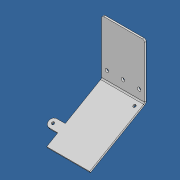
# Autodesk Inventor part: Fan_Holder
Saved by Autodesk Inventor 2020 (Build 240168000, 168)
## iProperties
Created: 2021-06-06
Part Number: Fan_Holder
Material: 一般
Document SubType Name: Sheet Metal
Designer: ken113
Density: 1 g/cm^3
Sheet Metal Rule: Default_mm
Appearance: 既定
Author: ken113
Autodesk Inventor part; units mm, degrees
ref_plane "YZ Plane" through (0, 0, 0) normal (1, 0, 0) x (0, 1, 0)
ref_plane "XZ Plane" through (0, 0, 0) normal (0, 1, 0) x (-1, 0, 0)
ref_plane "XY Plane" through (0, 0, 0) normal (0, 0, 1) x (1, 0, 0)
sketch "スケッチ1" plane through (0, 0, 0) normal (0, 0, 1) x (1, 0, 0)
  line L0 (20, 0) -> (-20, 0)
  line L1 (-20, 0) -> (-20, 50)
  line L2 (-20, 50) -> (20, 50)
  line L3 (20, 50) -> (20, 0)
  line L4 (20, 0) -> (-20, 50) construction
  line L5 (-20, 0) -> (20, 50) construction
  point P0 (0, 0)
  point P1 (0, 25)
  point P2 (0, 0)
  point P3 (0, 25)
  dimension "d0" = 40
  dimension "d1" = 50
  measures "d0" distance of L1.end L2.end
  measures "d1" distance of L0.end L1.end
extrude "プレート1" add sketch "スケッチ1" along normal blind 1.6
sketch "スケッチ2" plane through (20, -1.3856, 2.4) normal (0, -0.8660254, -0.5) x (1, 0, 0)
  line L0 (-40, 0) -> (0, 0)
  line L1 (0, 0) -> (0, 57.9525)
  line L2 (0, 57.9525) -> (-40, 57.9525)
  line L3 (-40, 57.9525) -> (-40, 0)
  constraints: 6 end point, 1 horizontal, 1 perpendicular, 1 vertical
edge flange "フランジ1" height 59.8 angle 60 thickness 1.6 bend radius 1.6 thickness toward (0, -0.8660254, -0.5) relief straight relief width 1.6 relief depth 0.8 edges at (0, 0, 1.6) wall of the first edge with corners at (-20, -1.3856, 2.4) (20, -1.3856, 2.4) (20, -30.3619, 52.5883) (-20, -30.3619, 52.5883)
bend "曲げ1"
corner "コーナー1"
sketch "スケッチ3" plane through (0, 0, 0) normal (0, 0, -1) x (-1, 0, 0)
  line L0 (-20, 0) -> (20, 0) projected
  line L1 (20, 0) -> (20, 50) projected
  line L2 (20, 50) -> (-20, 50) projected
  line L3 (-20, 50) -> (-20, 0) projected
  point P0 (0, 0)
  point P1 (-15, 8)
  point P2 (15, 8)
  point P3 (0, 8)
  point P4 (0, 0)
  dimension "d14" = 5
  dimension "d15" = 5
  dimension "d62" = 8
  constraints: 2 horizontal alignment, 1 midpoint, 1 vertical alignment
  measures "d14" distance from line of point (-15, 8) L3
  measures "d15" distance from line of L1 point (15, 8)
  measures "d62" distance from line of point (-15, 8) L0
hole "穴1" at (15, 8, 0) at (-15, 8, 0) at (0, 8, 0) direction (0, 0, 1) diameter 3.2 depth 1.6 tip angle 118
sketch "スケッチ4" plane through (-20, -31.7475, 51.7883) normal (0, -0.8660254, -0.5) x (1, 0, 0)
  line L0 (0, -57.9525) -> (40, -57.9525) projected
  line L1 (40, 0) -> (40, -57.9525) projected
  line L2 (0, 0) -> (40, 0) projected
  line L3 (0, -57.9525) -> (0, 0) projected
  point P0 (20, -60.7238)
  point P1 (35, -53.9525)
  dimension "d23" = 5
  dimension "d24" = 4
  measures "d23" distance from line of point (35, -53.952) L1
  measures "d24" distance from line of L0 point (35, -53.952)
hole "穴2" at (15, -4.7713, 5.0641) direction (0, 0.8660254, 0.5) diameter 2.459 end through all thread size "M3x0.5" class "6H" standard "ISO Metric profile"
sketch "スケッチ5" plane through (-20, -31.7475, 51.7883) normal (0, -0.8660254, -0.5) x (1, 0, 0)
  circle A0 centre (35, -53.9525) radius 1.2295 projected
  line L0 (0, 0) -> (0, -57.9525) projected
  line L1 (0, -11.9525) -> (-12, -11.9525)
  line L2 (-12, -11.9525) -> (-12, -19.9525)
  line L3 (-12, -19.9525) -> (0, -19.9525)
  line L4 (0, -19.9525) -> (0, -11.9525)
  point P0 (20, -60.7238)
  point P1 (-8, -15.9525)
  point P2 (0, -19.9525)
  dimension "d32" = 43
  dimension "d33" = 38
  dimension "d34" = 4
  dimension "d35" = 8
  dimension "d36" = 4
  constraints: 8 end point, 2 parallel, 1 horizontal, 1 perpendicular, 1 point on line
  measures "d32" horizontal distance of point (-8, -15.952) A0.centre
  measures "d33" vertical distance of point (-8, -15.952) A0.centre
  measures "d34" distance from line of point (-8, -15.952) L1
  measures "d35" distance of L1.end L2.end
  measures "d36" distance from line of point (-8, -15.952) L2
extrude "押し出し1" add sketch "スケッチ5" against normal up to surface (1.6 mm away) contours L0 L3 L2 L1
sketch "スケッチ6" plane through (-20, -31.7475, 51.7883) normal (0, -0.8660254, -0.5) x (1, 0, 0)
  circle A0 centre (35, -53.9525) radius 1.2295 projected
  point P0 (20, -60.7238)
  point P1 (-8, -15.9525)
  dimension "d39" = 43
  dimension "d40" = 38
  measures "d39" horizontal distance of point (-8, -15.952) A0.centre
  measures "d40" vertical distance of point (-8, -15.952) A0.centre
hole "穴3" at (-28, -23.7713, 37.9731) direction (0, 0.8660254, 0.5) diameter 2.459 depth 8.8 tip angle 118 thread size "M3x0.5" class "6H" standard "ISO Metric profile"
fillet "フィレット1" radius 4 2 edges at (-32, -21.0785, 34.909) (-32, -25.0785, 41.8372)
fillet "フィレット2" radius 2 2 edges at (20, 50, 0.8) (-20, 50, 0.8)
equation "\"d21\" = Thickness"
equation "\"d30\" = Thickness"
equation "\"d2\" = Thickness"
equation "\"d3\" = BendReliefWidth"
equation "\"d4\" = BendReliefDepth"
equation "\"d5\" = MinimumRemnant"
equation "\"d6\" = TransitionRadius"
equation "\"d9\" = BendRadius"
equation "\"d10\" = CornerReliefSize"
equation "\"d11\" = GapSize"
equation "\"d12\" = JacobiRadiusSize"
equation "\"BendRadius\" = Thickness"
equation "\"BendReliefWidth\" = Thickness"
equation "\"BendReliefDepth\" = 0.5 * Thickness"
equation "\"CornerReliefSize\" = 4 * Thickness"
equation "\"MinimumRemnant\" = 2 * Thickness"
equation "\"TransitionRadius\" = BendRadius"
equation "\"JacobiRadiusSize\" = BendRadius"
equation "\"GapSize\" = Thickness"
equation "\"Thickness\" = 1.6"
